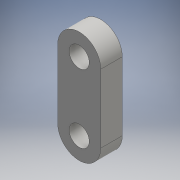
# Autodesk Inventor part: tracks_outer
Saved by Autodesk Inventor 2016 (Build 200138000, 138)
## iProperties
Created: 2016-05-02
Part Number: tracks_outer
Material: Generic
Document SubType Name: Modeling
Designer: Henrik Samuelsson
Density: 1 g/cm^3
Appearance: Default
Author: Henrik Samuelsson
Autodesk Inventor part; units mm, degrees
ref_plane "YZ Plane" through (0, 0, 0) normal (1, 0, 0) x (0, 1, 0)
ref_plane "XZ Plane" through (0, 0, 0) normal (0, 1, 0) x (-1, 0, 0)
ref_plane "XY Plane" through (0, 0, 0) normal (0, 0, 1) x (1, 0, 0)
sketch "Sketch1" plane through (0, 0, 0) normal (0, 1, 0) x (-1, 0, 0)
  line L0 (3, 0) -> (3, 0)
  line L1 (6, -3) -> (6, -12.525)
  line L2 (3, -15.525) -> (3, -15.525)
  line L3 (0, -12.525) -> (0, -3)
  arc A0 (6, -3) -> (3, 0) centre (3, -3) ccw
  arc A1 (3, 0) -> (0, -3) centre (3, -3) ccw
  arc A2 (3, -15.525) -> (6, -12.525) centre (3, -12.525) ccw
  arc A3 (0, -12.525) -> (3, -15.525) centre (3, -12.525) ccw
  circle A4 centre (3, -3) radius 1.4
  circle A5 centre (3, -12.525) radius 1.4
  point P0 (0, 0)
  point P1 (6, -15.525)
  point P2 (6, 0)
  point P3 (0, -15.525)
  dimension "d0" = 6
  dimension "d1" = 15.525
  dimension "d2" = 3
  dimension "d3" = 2.8
  dimension "d4" = 2.8
  constraints: 8 end point, 8 point on circle, 8 point on line, 8 tangent, 6 centre point, 3 equal radius, 2 coincident, 2 parallel, 1 horizontal, 1 perpendicular
  measures "d0" distance of point (6, -15.525) point (0, -15.525)
  measures "d1" distance of point (6, 0) point (6, -15.525)
  measures "d2" radius of A0
  measures "d3" diameter of A4
  measures "d4" diameter of A5
extrude "Extrusion1" add sketch "Sketch1" along normal blind 3
body "Solid1"
